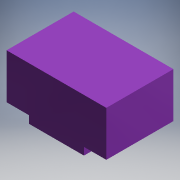
# Autodesk Inventor part: MPT4
Saved by Autodesk Inventor 2018.2 (Build 222227000, 227)
## iProperties
Part Number: MPT4
Material: Generic
Document SubType Name: Modeling
Designer: autocad
Appearance: 4POL254 NOPOL, MPT4
Author: autocad
Autodesk Inventor part; units mm, degrees
ref_plane "YZ Plane" through (0, 0, 0) normal (1, 0, 0) x (0, 1, 0)
ref_plane "XZ Plane" through (0, 0, 0) normal (0, 1, 0) x (-1, 0, 0)
ref_plane "XY Plane" through (0, 0, 0) normal (0, 0, 1) x (1, 0, 0)
sketch "4POL254 NOPOL, MPT4_183" plane through (0, 0, 0) normal (0, 0, 1) x (1, 0, 0)
  line L0 (-3.492, -2.857) -> (-6.3495, -2.857)
  line L1 (-6.3495, -2.857) -> (-6.3495, 2.8697)
  line L2 (-6.3495, 2.8697) -> (6.3495, 2.8697)
  line L3 (6.3495, 2.8697) -> (6.3495, -2.857)
  line L4 (6.3495, -2.857) -> (3.5047, -2.857)
  line L5 (3.5047, -2.857) -> (3.5047, -3.8095)
  line L6 (3.5047, -3.8095) -> (-3.492, -3.8095)
  line L7 (-3.492, -3.8095) -> (-3.492, -2.857)
  constraints: 16 end point
extrude "Extrusion1" add sketch "4POL254 NOPOL, MPT4_183" along normal blind 8.54
body "Solid1"
